Autodesk Fusion 360 part; units mm, degrees
(part 2 of 4)
  spline S9 degree 5 poles (13.0961, -23.3608) (13.1029, -23.373) (13.1162, -23.3975) (13.1351, -23.4347) (13.1584, -23.4852) (13.1848, -23.5497) (13.2094, -23.6151) (13.2328, -23.6811) (13.2556, -23.7474) (13.278, -23.814) (13.2999, -23.8807) (13.3212, -23.9477) (13.3416, -24.0151) (13.3612, -24.083) (13.3798, -24.1512) (13.3976, -24.2198) (13.4146, -24.2888) (13.4309, -24.358) (13.4467, -24.4275) (13.462, -24.4971) (13.4768, -24.567) (13.491, -24.6371) (13.5047, -24.7074) (13.5177, -24.778) (13.5302, -24.8488) (13.5421, -24.9198) (13.5534, -24.991) (13.5642, -25.0625) (13.5746, -25.1341) (13.5844, -25.2058) (13.5938, -25.2778) (13.6026, -25.3499) (13.611, -25.4222) (13.6189, -25.4947) (13.6263, -25.5673) (13.6332, -25.6401) (13.6397, -25.713) (13.6457, -25.7861) (13.6512, -25.8594) (13.6563, -25.9328) (13.661, -26.0063) (13.6652, -26.0799) (13.669, -26.1537) (13.6723, -26.2276) (13.6753, -26.3017) (13.6777, -26.3759) (13.6798, -26.4502) (13.6814, -26.5246) (13.6826, -26.5991) (13.6834, -26.6737) (13.6838, -26.7485) (13.6838, -26.8234) (13.6834, -26.8983) (13.6825, -26.9734) (13.6813, -27.0486) (13.6796, -27.1238) (13.6776, -27.1992) (13.6751, -27.2747) (13.6723, -27.3502) (13.6691, -27.4259) (13.6655, -27.5016) (13.6615, -27.5774) (13.6571, -27.6533) (13.6523, -27.7293) (13.6472, -27.8054) (13.6416, -27.8815) (13.6357, -27.9577) (13.6294, -28.034) (13.6228, -28.1104) (13.6157, -28.1868) (13.6083, -28.2633) (13.6021, -28.3246) (13.5973, -28.3705) (13.594, -28.4012) (13.5923, -28.4165) knots 0 0 0 0 0 0 0.01428571 0.02857143 0.04285714 0.05714286 0.07142857 0.08571429 0.1 0.11428571 0.12857143 0.14285714 0.15714286 0.17142857 0.18571429 0.2 0.21428571 0.22857143 0.24285714 0.25714286 0.27142857 0.28571429 0.3 0.31428571 0.32857143 0.34285714 0.35714286 0.37142857 0.38571429 0.4 0.41428571 0.42857143 0.44285714 0.45714286 0.47142857 0.48571429 0.5 0.51428571 0.52857143 0.54285714 0.55714286 0.57142857 0.58571429 0.6 0.61428571 0.62857143 0.64285714 0.65714286 0.67142857 0.68571429 0.7 0.71428571 0.72857143 0.74285714 0.75714286 0.77142857 0.78571429 0.8 0.81428571 0.82857143 0.84285714 0.85714286 0.87142857 0.88571429 0.9 0.91428571 0.92857143 0.94285714 0.95714286 0.97142857 0.98571429 1 1 1 1 1 1
  line L9 (13.0961, -23.3608) -> (12.631, -22.5302)
  arc A19 (12.9811, -21.189) -> (12.631, -22.5302) centre (13.5035, -22.0417) ccw
  arc A20 (12.9811, -21.189) -> (14.1898, -20.3993) centre (0, 0) ccw
  arc A21 (15.5588, -20.6174) -> (14.1898, -20.3993) centre (14.7609, -21.2202) ccw
  line L10 (15.5588, -20.6174) -> (16.1326, -21.377)
  spline S10 degree 5 poles (16.1326, -21.377) (16.141, -21.3881) (16.1581, -21.4101) (16.1845, -21.4424) (16.2215, -21.484) (16.2699, -21.5341) (16.3199, -21.5829) (16.371, -21.6309) (16.4225, -21.6784) (16.4745, -21.7256) (16.5268, -21.7724) (16.5797, -21.8189) (16.6332, -21.8647) (16.6874, -21.9098) (16.7424, -21.9543) (16.7981, -21.9981) (16.8545, -22.0414) (16.9113, -22.0842) (16.9685, -22.1266) (17.0262, -22.1686) (17.0842, -22.2102) (17.1427, -22.2513) (17.2016, -22.2921) (17.261, -22.3324) (17.3208, -22.3722) (17.3811, -22.4116) (17.4418, -22.4506) (17.5028, -22.4892) (17.5643, -22.5275) (17.626, -22.5653) (17.6882, -22.6028) (17.7507, -22.6399) (17.8135, -22.6766) (17.8767, -22.7129) (17.9402, -22.7489) (18.0041, -22.7845) (18.0683, -22.8197) (18.1328, -22.8545) (18.1977, -22.889) (18.2628, -22.9232) (18.3283, -22.957) (18.3941, -22.9904) (18.4601, -23.0235) (18.5265, -23.0563) (18.5931, -23.0887) (18.66, -23.1208) (18.7272, -23.1525) (18.7947, -23.1839) (18.8625, -23.2149) (18.9305, -23.2456) (18.9988, -23.276) (19.0674, -23.3061) (19.1362, -23.3358) (19.2053, -23.3652) (19.2746, -23.3942) (19.3442, -23.423) (19.4141, -23.4514) (19.4842, -23.4794) (19.5545, -23.5072) (19.6251, -23.5346) (19.6959, -23.5617) (19.7669, -23.5885) (19.8382, -23.615) (19.9097, -23.6412) (19.9814, -23.667) (20.0534, -23.6925) (20.1255, -23.7177) (20.1979, -23.7426) (20.2705, -23.7672) (20.3433, -23.7914) (20.4164, -23.8154) (20.475, -23.8343) (20.519, -23.8483) (20.5484, -23.8576) (20.5631, -23.8623) knots 0 0 0 0 0 0 0.01428571 0.02857143 0.04285714 0.05714286 0.07142857 0.08571429 0.1 0.11428571 0.12857143 0.14285714 0.15714286 0.17142857 0.18571429 0.2 0.21428571 0.22857143 0.24285714 0.25714286 0.27142857 0.28571429 0.3 0.31428571 0.32857143 0.34285714 0.35714286 0.37142857 0.38571429 0.4 0.41428571 0.42857143 0.44285714 0.45714286 0.47142857 0.48571429 0.5 0.51428571 0.52857143 0.54285714 0.55714286 0.57142857 0.58571429 0.6 0.61428571 0.62857143 0.64285714 0.65714286 0.67142857 0.68571429 0.7 0.71428571 0.72857143 0.74285714 0.75714286 0.77142857 0.78571429 0.8 0.81428571 0.82857143 0.84285714 0.85714286 0.87142857 0.88571429 0.9 0.91428571 0.92857143 0.94285714 0.95714286 0.97142857 0.98571429 1 1 1 1 1 1
  arc A22 (20.5631, -23.8623) -> (22.0827, -22.4634) centre (0, 0) ccw
  spline S11 degree 5 poles (19.9717, -17.8428) (19.9821, -17.8521) (20.0026, -17.8709) (20.0326, -17.9) (20.071, -17.9402) (20.117, -17.9926) (20.1615, -18.0465) (20.2051, -18.1013) (20.2482, -18.1566) (20.2909, -18.2123) (20.3333, -18.2683) (20.3752, -18.3248) (20.4165, -18.3819) (20.457, -18.4397) (20.4967, -18.4982) (20.5358, -18.5574) (20.5743, -18.6171) (20.6122, -18.6772) (20.6497, -18.7378) (20.6868, -18.7987) (20.7235, -18.86) (20.7597, -18.9217) (20.7955, -18.9837) (20.8307, -19.0463) (20.8655, -19.1092) (20.8998, -19.1725) (20.9336, -19.2362) (20.9671, -19.3002) (21.0001, -19.3646) (21.0327, -19.4293) (21.0649, -19.4943) (21.0967, -19.5596) (21.1281, -19.6253) (21.1591, -19.6913) (21.1897, -19.7576) (21.2199, -19.8241) (21.2497, -19.891) (21.2791, -19.9582) (21.3081, -20.0257) (21.3368, -20.0934) (21.365, -20.1615) (21.3929, -20.2298) (21.4205, -20.2983) (21.4476, -20.3672) (21.4744, -20.4362) (21.5009, -20.5056) (21.5269, -20.5752) (21.5526, -20.645) (21.578, -20.7151) (21.603, -20.7855) (21.6276, -20.8561) (21.6519, -20.9269) (21.6758, -20.9979) (21.6994, -21.0692) (21.7226, -21.1407) (21.7455, -21.2124) (21.7681, -21.2844) (21.7903, -21.3565) (21.8121, -21.4289) (21.8336, -21.5015) (21.8548, -21.5743) (21.8756, -21.6473) (21.8961, -21.7205) (21.9163, -21.7939) (21.9361, -21.8676) (21.9556, -21.9414) (21.9748, -22.0154) (21.9936, -22.0896) (22.0121, -22.164) (22.0302, -22.2385) (22.0481, -22.3133) (22.0621, -22.3733) (22.0724, -22.4183) (22.0793, -22.4484) (22.0827, -22.4634) knots 0 0 0 0 0 0 0.01428571 0.02857143 0.04285714 0.05714286 0.07142857 0.08571429 0.1 0.11428571 0.12857143 0.14285714 0.15714286 0.17142857 0.18571429 0.2 0.21428571 0.22857143 0.24285714 0.25714286 0.27142857 0.28571429 0.3 0.31428571 0.32857143 0.34285714 0.35714286 0.37142857 0.38571429 0.4 0.41428571 0.42857143 0.44285714 0.45714286 0.47142857 0.48571429 0.5 0.51428571 0.52857143 0.54285714 0.55714286 0.57142857 0.58571429 0.6 0.61428571 0.62857143 0.64285714 0.65714286 0.67142857 0.68571429 0.7 0.71428571 0.72857143 0.74285714 0.75714286 0.77142857 0.78571429 0.8 0.81428571 0.82857143 0.84285714 0.85714286 0.87142857 0.88571429 0.9 0.91428571 0.92857143 0.94285714 0.95714286 0.97142857 0.98571429 1 1 1 1 1 1
  line L11 (19.9717, -17.8428) -> (19.2622, -17.2082)
  arc A23 (19.1578, -15.8259) -> (19.2622, -17.2082) centre (19.9288, -16.4628) ccw
  arc A24 (19.1578, -15.8259) -> (20.0446, -14.6866) centre (0, 0) ccw
  arc A25 (21.4102, -14.4484) -> (20.0446, -14.6866) centre (20.8513, -15.2776) ccw
  line L12 (21.4102, -14.4484) -> (22.1996, -14.9805)
  spline S12 degree 5 poles (22.1996, -14.9805) (22.2111, -14.9883) (22.2344, -15.0035) (22.2699, -15.0254) (22.3184, -15.0528) (22.3805, -15.0845) (22.4436, -15.1144) (22.5075, -15.1432) (22.5717, -15.1714) (22.6361, -15.1992) (22.7008, -15.2265) (22.7659, -15.2532) (22.8314, -15.2792) (22.8974, -15.3043) (22.9638, -15.3285) (23.0308, -15.3519) (23.0981, -15.3745) (23.1657, -15.3965) (23.2336, -15.418) (23.3018, -15.439) (23.3702, -15.4595) (23.4389, -15.4795) (23.5078, -15.4989) (23.5771, -15.5177) (23.6466, -15.536) (23.7164, -15.5537) (23.7864, -15.5709) (23.8567, -15.5876) (23.9272, -15.6038) (23.998, -15.6195) (24.0689, -15.6348) (24.14, -15.6495) (24.2114, -15.6639) (24.283, -15.6777) (24.3547, -15.6911) (24.4267, -15.704) (24.4989, -15.7165) (24.5712, -15.7285) (24.6437, -15.7401) (24.7165, -15.7512) (24.7893, -15.7619) (24.8624, -15.7722) (24.9356, -15.7821) (25.009, -15.7915) (25.0826, -15.8005) (25.1563, -15.8091) (25.2302, -15.8173) (25.3042, -15.8251) (25.3783, -15.8324) (25.4527, -15.8394) (25.5271, -15.8459) (25.6017, -15.8521) (25.6765, -15.8579) (25.7514, -15.8632) (25.8264, -15.8682) (25.9015, -15.8728) (25.9768, -15.877) (26.0522, -15.8808) (26.1277, -15.8842) (26.2034, -15.8872) (26.2792, -15.8899) (26.3551, -15.8921) (26.4311, -15.894) (26.5072, -15.8956) (26.5834, -15.8967) (26.6598, -15.8975) (26.7362, -15.8979) (26.8127, -15.8979) (26.8894, -15.8976) (26.9662, -15.8969) (27.043, -15.8958) (27.1046, -15.8947) (27.1508, -15.8936) (27.1816, -15.8929) (27.197, -15.8925) knots 0 0 0 0 0 0 0.01428571 0.02857143 0.04285714 0.05714286 0.07142857 0.08571429 0.1 0.11428571 0.12857143 0.14285714 0.15714286 0.17142857 0.18571429 0.2 0.21428571 0.22857143 0.24285714 0.25714286 0.27142857 0.28571429 0.3 0.31428571 0.32857143 0.34285714 0.35714286 0.37142857 0.38571429 0.4 0.41428571 0.42857143 0.44285714 0.45714286 0.47142857 0.48571429 0.5 0.51428571 0.52857143 0.54285714 0.55714286 0.57142857 0.58571429 0.6 0.61428571 0.62857143 0.64285714 0.65714286 0.67142857 0.68571429 0.7 0.71428571 0.72857143 0.74285714 0.75714286 0.77142857 0.78571429 0.8 0.81428571 0.82857143 0.84285714 0.85714286 0.87142857 0.88571429 0.9 0.91428571 0.92857143 0.94285714 0.95714286 0.97142857 0.98571429 1 1 1 1 1 1
  arc A26 (27.197, -15.8925) -> (28.18, -14.0761) centre (0, 0) ccw
  spline S13 degree 5 poles (24.6832, -10.3912) (24.696, -10.3966) (24.7215, -10.4078) (24.7593, -10.4255) (24.8087, -10.4511) (24.8692, -10.4857) (24.9288, -10.5222) (24.9878, -10.5599) (25.0465, -10.5983) (25.105, -10.6371) (25.1633, -10.6763) (25.2213, -10.7161) (25.2788, -10.7567) (25.3359, -10.7982) (25.3925, -10.8407) (25.4487, -10.8839) (25.5045, -10.9279) (25.5599, -10.9725) (25.615, -11.0175) (25.6699, -11.0631) (25.7245, -11.1092) (25.7787, -11.1558) (25.8327, -11.2029) (25.8863, -11.2506) (25.9397, -11.2988) (25.9927, -11.3475) (26.0454, -11.3968) (26.0978, -11.4465) (26.1499, -11.4966) (26.2018, -11.5472) (26.2533, -11.5983) (26.3046, -11.6497) (26.3556, -11.7016) (26.4064, -11.754) (26.4568, -11.8068) (26.507, -11.8599) (26.5569, -11.9135) (26.6065, -11.9675) (26.6559, -12.0219) (26.705, -12.0767) (26.7538, -12.1318) (26.8024, -12.1874) (26.8507, -12.2433) (26.8988, -12.2996) (26.9465, -12.3562) (26.994, -12.4132) (27.0413, -12.4706) (27.0883, -12.5283) (27.135, -12.5864) (27.1815, -12.6448) (27.2277, -12.7035) (27.2737, -12.7626) (27.3194, -12.8221) (27.3648, -12.8818) (27.41, -12.9419) (27.455, -13.0023) (27.4996, -13.063) (27.5441, -13.1241) (27.5882, -13.1855) (27.6321, -13.2471) (27.6758, -13.3091) (27.7192, -13.3714) (27.7624, -13.434) (27.8053, -13.4969) (27.8479, -13.5601) (27.8903, -13.6236) (27.9325, -13.6873) (27.9744, -13.7514) (28.016, -13.8158) (28.0574, -13.8804) (28.0986, -13.9453) (28.1313, -13.9975) (28.1557, -14.0367) (28.1719, -14.063) (28.18, -14.0761) knots 0 0 0 0 0 0 0.01428571 0.02857143 0.04285714 0.05714286 0.07142857 0.08571429 0.1 0.11428571 0.12857143 0.14285714 0.15714286 0.17142857 0.18571429 0.2 0.21428571 0.22857143 0.24285714 0.25714286 0.27142857 0.28571429 0.3 0.31428571 0.32857143 0.34285714 0.35714286 0.37142857 0.38571429 0.4 0.41428571 0.42857143 0.44285714 0.45714286 0.47142857 0.48571429 0.5 0.51428571 0.52857143 0.54285714 0.55714286 0.57142857 0.58571429 0.6 0.61428571 0.62857143 0.64285714 0.65714286 0.67142857 0.68571429 0.7 0.71428571 0.72857143 0.74285714 0.75714286 0.77142857 0.78571429 0.8 0.81428571 0.82857143 0.84285714 0.85714286 0.87142857 0.88571429 0.9 0.91428571 0.92857143 0.94285714 0.95714286 0.97142857 0.98571429 1 1 1 1 1 1
  line L13 (24.6832, -10.3912) -> (23.806, -10.0214)
  arc A27 (23.2585, -8.7479) -> (23.806, -10.0214) centre (24.1945, -9.0999) ccw
  arc A28 (23.2585, -8.7479) -> (23.7273, -7.3823) centre (0, 0) ccw
  arc A29 (24.9416, -6.7137) -> (23.7273, -7.3823) centre (24.6821, -7.6794) ccw
  line L14 (24.9416, -6.7137) -> (25.8609, -6.9606)
  spline S14 degree 5 poles (25.8609, -6.9606) (25.8743, -6.9642) (25.9013, -6.9711) (25.942, -6.9803) (25.9968, -6.9904) (26.0658, -7.0003) (26.1352, -7.008) (26.2049, -7.0145) (26.2748, -7.0204) (26.3448, -7.0257) (26.4149, -7.0305) (26.4851, -7.0347) (26.5555, -7.038) (26.626, -7.0403) (26.6967, -7.0416) (26.7676, -7.042) (26.8386, -7.0415) (26.9098, -7.0404) (26.981, -7.0387) (27.0523, -7.0364) (27.1236, -7.0336) (27.1951, -7.0302) (27.2666, -7.0261) (27.3382, -7.0215) (27.4099, -7.0161) (27.4817, -7.0102) (27.5535, -7.0037) (27.6254, -6.9967) (27.6973, -6.9891) (27.7693, -6.9811) (27.8414, -6.9725) (27.9135, -6.9634) (27.9856, -6.9537) (28.0578, -6.9436) (28.13, -6.9329) (28.2023, -6.9218) (28.2746, -6.9101) (28.3469, -6.898) (28.4193, -6.8854) (28.4917, -6.8723) (28.5641, -6.8588) (28.6365, -6.8448) (28.709, -6.8304) (28.7814, -6.8155) (28.8539, -6.8001) (28.9265, -6.7843) (28.999, -6.7681) (29.0715, -6.7514) (29.1441, -6.7343) (29.2166, -6.7167) (29.2892, -6.6987) (29.3617, -6.6803) (29.4343, -6.6615) (29.5069, -6.6423) (29.5794, -6.6226) (29.652, -6.6025) (29.7246, -6.582) (29.7971, -6.5612) (29.8697, -6.5399) (29.9422, -6.5182) (30.0147, -6.4961) (30.0872, -6.4736) (30.1597, -6.4507) (30.2322, -6.4274) (30.3047, -6.4038) (30.3772, -6.3797) (30.4496, -6.3553) (30.522, -6.3304) (30.5944, -6.3052) (30.6668, -6.2796) (30.7391, -6.2537) (30.797, -6.2326) (30.8403, -6.2166) (30.8693, -6.2059) (30.8837, -6.2005) knots 0 0 0 0 0 0 0.01428571 0.02857143 0.04285714 0.05714286 0.07142857 0.08571429 0.1 0.11428571 0.12857143 0.14285714 0.15714286 0.17142857 0.18571429 0.2 0.21428571 0.22857143 0.24285714 0.25714286 0.27142857 0.28571429 0.3 0.31428571 0.32857143 0.34285714 0.35714286 0.37142857 0.38571429 0.4 0.41428571 0.42857143 0.44285714 0.45714286 0.47142857 0.48571429 0.5 0.51428571 0.52857143 0.54285714 0.55714286 0.57142857 0.58571429 0.6 0.61428571 0.62857143 0.64285714 0.65714286 0.67142857 0.68571429 0.7 0.71428571 0.72857143 0.74285714 0.75714286 0.77142857 0.78571429 0.8 0.81428571 0.82857143 0.84285714 0.85714286 0.87142857 0.88571429 0.9 0.91428571 0.92857143 0.94285714 0.95714286 0.97142857 0.98571429 1 1 1 1 1 1
  arc A30 (30.8837, -6.2005) -> (31.2237, -4.1634) centre (0, 0) ccw
  spline S15 degree 5 poles (26.7198, -1.8136) (26.7337, -1.8145) (26.7614, -1.8168) (26.8029, -1.8213) (26.858, -1.8295) (26.9264, -1.8426) (26.9947, -1.8578) (27.0627, -1.8742) (27.1307, -1.8914) (27.1986, -1.9091) (27.2665, -1.9273) (27.3342, -1.9461) (27.4019, -1.9659) (27.4693, -1.9866) (27.5366, -2.0083) (27.6038, -2.031) (27.6708, -2.0545) (27.7377, -2.0787) (27.8045, -2.1034) (27.8712, -2.1287) (27.9378, -2.1545) (28.0043, -2.181) (28.0706, -2.208) (28.1368, -2.2357) (28.2029, -2.264) (28.2688, -2.2929) (28.3347, -2.3223) (28.4004, -2.3523) (28.466, -2.3829) (28.5315, -2.4139) (28.5968, -2.4454) (28.662, -2.4774) (28.7271, -2.51) (28.7921, -2.543) (28.857, -2.5765) (28.9217, -2.6105) (28.9863, -2.645) (29.0508, -2.68) (29.1151, -2.7154) (29.1794, -2.7512) (29.2434, -2.7876) (29.3074, -2.8243) (29.3713, -2.8615) (29.435, -2.8991) (29.4986, -2.9372) (29.562, -2.9757) (29.6253, -3.0146) (29.6885, -3.0539) (29.7516, -3.0937) (29.8145, -3.1338) (29.8773, -3.1744) (29.9399, -3.2154) (30.0025, -3.2567) (30.0648, -3.2985) (30.1271, -3.3407) (30.1892, -3.3832) (30.2512, -3.4261) (30.313, -3.4695) (30.3747, -3.5131) (30.4363, -3.5572) (30.4977, -3.6017) (30.559, -3.6465) (30.6201, -3.6917) (30.6811, -3.7372) (30.742, -3.7831) (30.8027, -3.8294) (30.8633, -3.8761) (30.9237, -3.923) (30.984, -3.9704) (31.0441, -4.0181) (31.1041, -4.0661) (31.152, -4.1049) (31.1879, -4.134) (31.2117, -4.1536) (31.2237, -4.1634) knots 0 0 0 0 0 0 0.01428571 0.02857143 0.04285714 0.05714286 0.07142857 0.08571429 0.1 0.11428571 0.12857143 0.14285714 0.15714286 0.17142857 0.18571429 0.2 0.21428571 0.22857143 0.24285714 0.25714286 0.27142857 0.28571429 0.3 0.31428571 0.32857143 0.34285714 0.35714286 0.37142857 0.38571429 0.4 0.41428571 0.42857143 0.44285714 0.45714286 0.47142857 0.48571429 0.5 0.51428571 0.52857143 0.54285714 0.55714286 0.57142857 0.58571429 0.6 0.61428571 0.62857143 0.64285714 0.65714286 0.67142857 0.68571429 0.7 0.71428571 0.72857143 0.74285714 0.75714286 0.77142857 0.78571429 0.8 0.81428571 0.82857143 0.84285714 0.85714286 0.87142857 0.88571429 0.9 0.91428571 0.92857143 0.94285714 0.95714286 0.97142857 0.98571429 1 1 1 1 1 1
  line L15 (26.7198, -1.8136) -> (25.7701, -1.7486)
  arc A31 (24.8387, -0.7219) -> (25.7701, -1.7486) centre (25.8383, -0.7509) ccw
  arc A32 (24.8387, -0.7219) -> (24.8387, 0.7219) centre (0, 0) ccw
  arc A33 (25.7701, 1.7486) -> (24.8387, 0.7219) centre (25.8383, 0.7509) ccw
  line L16 (25.7701, 1.7486) -> (26.7198, 1.8136)
  spline S16 degree 5 poles (26.7198, 1.8136) (26.7337, 1.8145) (26.7614, 1.8168) (26.8029, 1.8213) (26.858, 1.8295) (26.9264, 1.8426) (26.9947, 1.8578) (27.0627, 1.8742) (27.1307, 1.8914) (27.1986, 1.9091) (27.2665, 1.9273) (27.3342, 1.9461) (27.4019, 1.9659) (27.4693, 1.9866) (27.5366, 2.0083) (27.6038, 2.031) (27.6708, 2.0545) (27.7377, 2.0787) (27.8045, 2.1034) (27.8712, 2.1287) (27.9378, 2.1545) (28.0043, 2.181) (28.0706, 2.208) (28.1368, 2.2357) (28.2029, 2.264) (28.2688, 2.2929) (28.3347, 2.3223) (28.4004, 2.3523) (28.466, 2.3829) (28.5315, 2.4139) (28.5968, 2.4454) (28.662, 2.4774) (28.7271, 2.51) (28.7921, 2.543) (28.857, 2.5765) (28.9217, 2.6105) (28.9863, 2.645) (29.0508, 2.68) (29.1151, 2.7154) (29.1794, 2.7512) (29.2434, 2.7876) (29.3074, 2.8243) (29.3713, 2.8615) (29.435, 2.8991) (29.4986, 2.9372) (29.562, 2.9757) (29.6253, 3.0146) (29.6885, 3.0539) (29.7516, 3.0937) (29.8145, 3.1338) (29.8773, 3.1744) (29.9399, 3.2154) (30.0025, 3.2567) (30.0648, 3.2985) (30.1271, 3.3407) (30.1892, 3.3832) (30.2512, 3.4261) (30.313, 3.4695) (30.3747, 3.5131) (30.4363, 3.5572) (30.4977, 3.6017) (30.559, 3.6465) (30.6201, 3.6917) (30.6811, 3.7372) (30.742, 3.7831) (30.8027, 3.8294) (30.8633, 3.8761) (30.9237, 3.923) (30.984, 3.9704) (31.0441, 4.0181) (31.1041, 4.0661) (31.152, 4.1049) (31.1879, 4.134) (31.2117, 4.1536) (31.2237, 4.1634) knots 0 0 0 0 0 0 0.01428571 0.02857143 0.04285714 0.05714286 0.07142857 0.08571429 0.1 0.11428571 0.12857143 0.14285714 0.15714286 0.17142857 0.18571429 0.2 0.21428571 0.22857143 0.24285714 0.25714286 0.27142857 0.28571429 0.3 0.31428571 0.32857143 0.34285714 0.35714286 0.37142857 0.38571429 0.4 0.41428571 0.42857143 0.44285714 0.45714286 0.47142857 0.48571429 0.5 0.51428571 0.52857143 0.54285714 0.55714286 0.57142857 0.58571429 0.6 0.61428571 0.62857143 0.64285714 0.65714286 0.67142857 0.68571429 0.7 0.71428571 0.72857143 0.74285714 0.75714286 0.77142857 0.78571429 0.8 0.81428571 0.82857143 0.84285714 0.85714286 0.87142857 0.88571429 0.9 0.91428571 0.92857143 0.94285714 0.95714286 0.97142857 0.98571429 1 1 1 1 1 1
  arc A34 (31.2237, 4.1634) -> (30.8837, 6.2005) centre (0, 0) ccw
  spline S17 degree 5 poles (25.8609, 6.9606) (25.8743, 6.9642) (25.9013, 6.9711) (25.942, 6.9803) (25.9968, 6.9904) (26.0658, 7.0003) (26.1352, 7.008) (26.2049, 7.0145) (26.2748, 7.0204) (26.3448, 7.0257) (26.4149, 7.0305) (26.4851, 7.0347) (26.5555, 7.038) (26.626, 7.0403) (26.6967, 7.0416) (26.7676, 7.042) (26.8386, 7.0415) (26.9098, 7.0404) (26.981, 7.0387) (27.0523, 7.0364) (27.1236, 7.0336) (27.1951, 7.0302) (27.2666, 7.0261) (27.3382, 7.0215) (27.4099, 7.0161) (27.4817, 7.0102) (27.5535, 7.0037) (27.6254, 6.9967) (27.6973, 6.9891) (27.7693, 6.9811) (27.8414, 6.9725) (27.9135, 6.9634) (27.9856, 6.9537) (28.0578, 6.9436) (28.13, 6.9329) (28.2023, 6.9218) (28.2746, 6.9101) (28.3469, 6.898) (28.4193, 6.8854) (28.4917, 6.8723) (28.5641, 6.8588) (28.6365, 6.8448) (28.709, 6.8304) (28.7814, 6.8155) (28.8539, 6.8001) (28.9265, 6.7843) (28.999, 6.7681) (29.0715, 6.7514) (29.1441, 6.7343) (29.2166, 6.7167) (29.2892, 6.6987) (29.3617, 6.6803) (29.4343, 6.6615) (29.5069, 6.6423) (29.5794, 6.6226) (29.652, 6.6025) (29.7246, 6.582) (29.7971, 6.5612) (29.8697, 6.5399) (29.9422, 6.5182) (30.0147, 6.4961) (30.0872, 6.4736) (30.1597, 6.4507) (30.2322, 6.4274) (30.3047, 6.4038) (30.3772, 6.3797) (30.4496, 6.3553) (30.522, 6.3304) (30.5944, 6.3052) (30.6668, 6.2796) (30.7391, 6.2537) (30.797, 6.2326) (30.8403, 6.2166) (30.8693, 6.2059) (30.8837, 6.2005) knots 0 0 0 0 0 0 0.01428571 0.02857143 0.04285714 0.05714286 0.07142857 0.08571429 0.1 0.11428571 0.12857143 0.14285714 0.15714286 0.17142857 0.18571429 0.2 0.21428571 0.22857143 0.24285714 0.25714286 0.27142857 0.28571429 0.3 0.31428571 0.32857143 0.34285714 0.35714286 0.37142857 0.38571429 0.4 0.41428571 0.42857143 0.44285714 0.45714286 0.47142857 0.48571429 0.5 0.51428571 0.52857143 0.54285714 0.55714286 0.57142857 0.58571429 0.6 0.61428571 0.62857143 0.64285714 0.65714286 0.67142857 0.68571429 0.7 0.71428571 0.72857143 0.74285714 0.75714286 0.77142857 0.78571429 0.8 0.81428571 0.82857143 0.84285714 0.85714286 0.87142857 0.88571429 0.9 0.91428571 0.92857143 0.94285714 0.95714286 0.97142857 0.98571429 1 1 1 1 1 1
  line L17 (25.8609, 6.9606) -> (24.9416, 6.7137)
  arc A35 (23.7273, 7.3823) -> (24.9416, 6.7137) centre (24.6821, 7.6794) ccw
  arc A36 (23.7273, 7.3823) -> (23.2585, 8.7479) centre (0, 0) ccw
  arc A37 (23.806, 10.0214) -> (23.2585, 8.7479) centre (24.1945, 9.0999) ccw
  line L18 (23.806, 10.0214) -> (24.6832, 10.3912)
  spline S18 degree 5 poles (24.6832, 10.3912) (24.696, 10.3966) (24.7215, 10.4078) (24.7593, 10.4255) (24.8087, 10.4511) (24.8692, 10.4857) (24.9288, 10.5222) (24.9878, 10.5599) (25.0465, 10.5983) (25.105, 10.6371) (25.1633, 10.6763) (25.2213, 10.7161) (25.2788, 10.7567) (25.3359, 10.7982) (25.3925, 10.8407) (25.4487, 10.8839) (25.5045, 10.9279) (25.5599, 10.9725) (25.615, 11.0175) (25.6699, 11.0631) (25.7245, 11.1092) (25.7787, 11.1558) (25.8327, 11.2029) (25.8863, 11.2506) (25.9397, 11.2988) (25.9927, 11.3475) (26.0454, 11.3968) (26.0978, 11.4465) (26.1499, 11.4966) (26.2018, 11.5472) (26.2533, 11.5983) (26.3046, 11.6497) (26.3556, 11.7016) (26.4064, 11.754) (26.4568, 11.8068) (26.507, 11.8599) (26.5569, 11.9135) (26.6065, 11.9675) (26.6559, 12.0219) (26.705, 12.0767) (26.7538, 12.1318) (26.8024, 12.1874) (26.8507, 12.2433) (26.8988, 12.2996) (26.9465, 12.3562) (26.994, 12.4132) (27.0413, 12.4706) (27.0883, 12.5283) (27.135, 12.5864) (27.1815, 12.6448) (27.2277, 12.7035) (27.2737, 12.7626) (27.3194, 12.8221) (27.3648, 12.8818) (27.41, 12.9419) (27.455, 13.0023) (27.4996, 13.063) (27.5441, 13.1241) (27.5882, 13.1855) (27.6321, 13.2471) (27.6758, 13.3091) (27.7192, 13.3714) (27.7624, 13.434) (27.8053, 13.4969) (27.8479, 13.5601) (27.8903, 13.6236) (27.9325, 13.6873) (27.9744, 13.7514) (28.016, 13.8158) (28.0574, 13.8804) (28.0986, 13.9453) (28.1313, 13.9975) (28.1557, 14.0367) (28.1719, 14.063) (28.18, 14.0761) knots 0 0 0 0 0 0 0.01428571 0.02857143 0.04285714 0.05714286 0.07142857 0.08571429 0.1 0.11428571 0.12857143 0.14285714 0.15714286 0.17142857 0.18571429 0.2 0.21428571 0.22857143 0.24285714 0.25714286 0.27142857 0.28571429 0.3 0.31428571 0.32857143 0.34285714 0.35714286 0.37142857 0.38571429 0.4 0.41428571 0.42857143 0.44285714 0.45714286 0.47142857 0.48571429 0.5 0.51428571 0.52857143 0.54285714 0.55714286 0.57142857 0.58571429 0.6 0.61428571 0.62857143 0.64285714 0.65714286 0.67142857 0.68571429 0.7 0.71428571 0.72857143 0.74285714 0.75714286 0.77142857 0.78571429 0.8 0.81428571 0.82857143 0.84285714 0.85714286 0.87142857 0.88571429 0.9 0.91428571 0.92857143 0.94285714 0.95714286 0.97142857 0.98571429 1 1 1 1 1 1
  arc A38 (28.18, 14.0761) -> (27.197, 15.8925) centre (0, 0) ccw
  spline S19 degree 5 poles (22.1996, 14.9805) (22.2111, 14.9883) (22.2344, 15.0035) (22.2699, 15.0254) (22.3184, 15.0528) (22.3805, 15.0845) (22.4436, 15.1144) (22.5075, 15.1432) (22.5717, 15.1714) (22.6361, 15.1992) (22.7008, 15.2265) (22.7659, 15.2532) (22.8314, 15.2792) (22.8974, 15.3043) (22.9638, 15.3285) (23.0308, 15.3519) (23.0981, 15.3745) (23.1657, 15.3965) (23.2336, 15.418) (23.3018, 15.439) (23.3702, 15.4595) (23.4389, 15.4795) (23.5078, 15.4989) (23.5771, 15.5177) (23.6466, 15.536) (23.7164, 15.5537) (23.7864, 15.5709) (23.8567, 15.5876) (23.9272, 15.6038) (23.998, 15.6195) (24.0689, 15.6348) (24.14, 15.6495) (24.2114, 15.6639) (24.283, 15.6777) (24.3547, 15.6911) (24.4267, 15.704) (24.4989, 15.7165) (24.5712, 15.7285) (24.6437, 15.7401) (24.7165, 15.7512) (24.7893, 15.7619) (24.8624, 15.7722) (24.9356, 15.7821) (25.009, 15.7915) (25.0826, 15.8005) (25.1563, 15.8091) (25.2302, 15.8173) (25.3042, 15.8251) (25.3783, 15.8324) (25.4527, 15.8394) (25.5271, 15.8459) (25.6017, 15.8521) (25.6765, 15.8579) (25.7514, 15.8632) (25.8264, 15.8682) (25.9015, 15.8728) (25.9768, 15.877) (26.0522, 15.8808) (26.1277, 15.8842) (26.2034, 15.8872) (26.2792, 15.8899) (26.3551, 15.8921) (26.4311, 15.894) (26.5072, 15.8956) (26.5834, 15.8967) (26.6598, 15.8975) (26.7362, 15.8979) (26.8127, 15.8979) (26.8894, 15.8976) (26.9662, 15.8969) (27.043, 15.8958) (27.1046, 15.8947) (27.1508, 15.8936) (27.1816, 15.8929) (27.197, 15.8925) knots 0 0 0 0 0 0 0.01428571 0.02857143 0.04285714 0.05714286 0.07142857 0.08571429 0.1 0.11428571 0.12857143 0.14285714 0.15714286 0.17142857 0.18571429 0.2 0.21428571 0.22857143 0.24285714 0.25714286 0.27142857 0.28571429 0.3 0.31428571 0.32857143 0.34285714 0.35714286 0.37142857 0.38571429 0.4 0.41428571 0.42857143 0.44285714 0.45714286 0.47142857 0.48571429 0.5 0.51428571 0.52857143 0.54285714 0.55714286 0.57142857 0.58571429 0.6 0.61428571 0.62857143 0.64285714 0.65714286 0.67142857 0.68571429 0.7 0.71428571 0.72857143 0.74285714 0.75714286 0.77142857 0.78571429 0.8 0.81428571 0.82857143 0.84285714 0.85714286 0.87142857 0.88571429 0.9 0.91428571 0.92857143 0.94285714 0.95714286 0.97142857 0.98571429 1 1 1 1 1 1
  line L19 (22.1996, 14.9805) -> (21.4102, 14.4484)
  arc A39 (20.0446, 14.6866) -> (21.4102, 14.4484) centre (20.8513, 15.2776) ccw
  arc A40 (20.0446, 14.6866) -> (19.1578, 15.8259) centre (0, 0) ccw
  arc A41 (19.2622, 17.2082) -> (19.1578, 15.8259) centre (19.9288, 16.4628) ccw
  line L20 (19.2622, 17.2082) -> (19.9717, 17.8428)
  spline S20 degree 5 poles (19.9717, 17.8428) (19.9821, 17.8521) (20.0026, 17.8709) (20.0326, 17.9) (20.071, 17.9402) (20.117, 17.9926) (20.1615, 18.0465) (20.2051, 18.1013) (20.2482, 18.1566) (20.2909, 18.2123) (20.3333, 18.2683) (20.3752, 18.3248) (20.4165, 18.3819) (20.457, 18.4397) (20.4967, 18.4982) (20.5358, 18.5574) (20.5743, 18.6171) (20.6122, 18.6772) (20.6497, 18.7378) (20.6868, 18.7987) (20.7235, 18.86) (20.7597, 18.9217) (20.7955, 18.9837) (20.8307, 19.0463) (20.8655, 19.1092) (20.8998, 19.1725) (20.9336, 19.2362) (20.9671, 19.3002) (21.0001, 19.3646) (21.0327, 19.4293) (21.0649, 19.4943) (21.0967, 19.5596) (21.1281, 19.6253) (21.1591, 19.6913) (21.1897, 19.7576) (21.2199, 19.8241) (21.2497, 19.891) (21.2791, 19.9582) (21.3081, 20.0257) (21.3368, 20.0934) (21.365, 20.1615) (21.3929, 20.2298) (21.4205, 20.2983) (21.4476, 20.3672) (21.4744, 20.4362) (21.5009, 20.5056) (21.5269, 20.5752) (21.5526, 20.645) (21.578, 20.7151) (21.603, 20.7855) (21.6276, 20.8561) (21.6519, 20.9269) (21.6758, 20.9979) (21.6994, 21.0692) (21.7226, 21.1407) (21.7455, 21.2124) (21.7681, 21.2844) (21.7903, 21.3565) (21.8121, 21.4289) (21.8336, 21.5015) (21.8548, 21.5743) (21.8756, 21.6473) (21.8961, 21.7205) (21.9163, 21.7939) (21.9361, 21.8676) (21.9556, 21.9414) (21.9748, 22.0154) (21.9936, 22.0896) (22.0121, 22.164) (22.0302, 22.2385) (22.0481, 22.3133) (22.0621, 22.3733) (22.0724, 22.4183) (22.0793, 22.4484) (22.0827, 22.4634) knots 0 0 0 0 0 0 0.01428571 0.02857143 0.04285714 0.05714286 0.07142857 0.08571429 0.1 0.11428571 0.12857143 0.14285714 0.15714286 0.17142857 0.18571429 0.2 0.21428571 0.22857143 0.24285714 0.25714286 0.27142857 0.28571429 0.3 0.31428571 0.32857143 0.34285714 0.35714286 0.37142857 0.38571429 0.4 0.41428571 0.42857143 0.44285714 0.45714286 0.47142857 0.48571429 0.5 0.51428571 0.52857143 0.54285714 0.55714286 0.57142857 0.58571429 0.6 0.61428571 0.62857143 0.64285714 0.65714286 0.67142857 0.68571429 0.7 0.71428571 0.72857143 0.74285714 0.75714286 0.77142857 0.78571429 0.8 0.81428571 0.82857143 0.84285714 0.85714286 0.87142857 0.88571429 0.9 0.91428571 0.92857143 0.94285714 0.95714286 0.97142857 0.98571429 1 1 1 1 1 1
  arc A42 (22.0827, 22.4634) -> (20.5631, 23.8623) centre (0, 0) ccw
  spline S21 degree 5 poles (16.1326, 21.377) (16.141, 21.3881) (16.1581, 21.4101) (16.1845, 21.4424) (16.2215, 21.484) (16.2699, 21.5341) (16.3199, 21.5829) (16.371, 21.6309) (16.4225, 21.6784) (16.4745, 21.7256) (16.5268, 21.7724) (16.5797, 21.8189) (16.6332, 21.8647) (16.6874, 21.9098) (16.7424, 21.9543) (16.7981, 21.9981) (16.8545, 22.0414) (16.9113, 22.0842) (16.9685, 22.1266) (17.0262, 22.1686) (17.0842, 22.2102) (17.1427, 22.2513) (17.2016, 22.2921) (17.261, 22.3324) (17.3208, 22.3722) (17.3811, 22.4116) (17.4418, 22.4506) (17.5028, 22.4892) (17.5643, 22.5275) (17.626, 22.5653) (17.6882, 22.6028) (17.7507, 22.6399) (17.8135, 22.6766) (17.8767, 22.7129) (17.9402, 22.7489) (18.0041, 22.7845) (18.0683, 22.8197) (18.1328, 22.8545) (18.1977, 22.889) (18.2628, 22.9232) (18.3283, 22.957) (18.3941, 22.9904) (18.4601, 23.0235) (18.5265, 23.0563) (18.5931, 23.0887) (18.66, 23.1208) (18.7272, 23.1525) (18.7947, 23.1839) (18.8625, 23.2149) (18.9305, 23.2456) (18.9988, 23.276) (19.0674, 23.3061) (19.1362, 23.3358) (19.2053, 23.3652) (19.2746, 23.3942) (19.3442, 23.423) (19.4141, 23.4514) (19.4842, 23.4794) (19.5545, 23.5072) (19.6251, 23.5346) (19.6959, 23.5617) (19.7669, 23.5885) (19.8382, 23.615) (19.9097, 23.6412) (19.9814, 23.667) (20.0534, 23.6925) (20.1255, 23.7177) (20.1979, 23.7426) (20.2705, 23.7672) (20.3433, 23.7914) (20.4164, 23.8154) (20.475, 23.8343) (20.519, 23.8483) (20.5484, 23.8576) (20.5631, 23.8623) knots 0 0 0 0 0 0 0.01428571 0.02857143 0.04285714 0.05714286 0.07142857 0.08571429 0.1 0.11428571 0.12857143 0.14285714 0.15714286 0.17142857 0.18571429 0.2 0.21428571 0.22857143 0.24285714 0.25714286 0.27142857 0.28571429 0.3 0.31428571 0.32857143 0.34285714 0.35714286 0.37142857 0.38571429 0.4 0.41428571 0.42857143 0.44285714 0.45714286 0.47142857 0.48571429 0.5 0.51428571 0.52857143 0.54285714 0.55714286 0.57142857 0.58571429 0.6 0.61428571 0.62857143 0.64285714 0.65714286 0.67142857 0.68571429 0.7 0.71428571 0.72857143 0.74285714 0.75714286 0.77142857 0.78571429 0.8 0.81428571 0.82857143 0.84285714 0.85714286 0.87142857 0.88571429 0.9 0.91428571 0.92857143 0.94285714 0.95714286 0.97142857 0.98571429 1 1 1 1 1 1
  line L21 (16.1326, 21.377) -> (15.5588, 20.6174)
  arc A43 (14.1898, 20.3993) -> (15.5588, 20.6174) centre (14.7609, 21.2202) ccw
  arc A44 (14.1898, 20.3993) -> (12.9811, 21.189) centre (0, 0) ccw
  arc A45 (12.631, 22.5302) -> (12.9811, 21.189) centre (13.5035, 22.0417) ccw
  line L22 (12.631, 22.5302) -> (13.0961, 23.3608)
  spline S22 degree 5 poles (13.0961, 23.3608) (13.1029, 23.373) (13.1162, 23.3975) (13.1351, 23.4347) (13.1584, 23.4852) (13.1848, 23.5497) (13.2094, 23.6151) (13.2328, 23.6811) (13.2556, 23.7474) (13.278, 23.814) (13.2999, 23.8807) (13.3212, 23.9477) (13.3416, 24.0151) (13.3612, 24.083) (13.3798, 24.1512) (13.3976, 24.2198) (13.4146, 24.2888) (13.4309, 24.358) (13.4467, 24.4275) (13.462, 24.4971) (13.4768, 24.567) (13.491, 24.6371) (13.5047, 24.7074) (13.5177, 24.778) (13.5302, 24.8488) (13.5421, 24.9198) (13.5534, 24.991) (13.5642, 25.0625) (13.5746, 25.1341) (13.5844, 25.2058) (13.5938, 25.2778) (13.6026, 25.3499) (13.611, 25.4222) (13.6189, 25.4947) (13.6263, 25.5673) (13.6332, 25.6401) (13.6397, 25.713) (13.6457, 25.7861) (13.6512, 25.8594) (13.6563, 25.9328) (13.661, 26.0063) (13.6652, 26.0799) (13.669, 26.1537) (13.6723, 26.2276) (13.6753, 26.3017) (13.6777, 26.3759) (13.6798, 26.4502) (13.6814, 26.5246) (13.6826, 26.5991) (13.6834, 26.6737) (13.6838, 26.7485) (13.6838, 26.8234) (13.6834, 26.8983) (13.6825, 26.9734) (13.6813, 27.0486) (13.6796, 27.1238) (13.6776, 27.1992) (13.6751, 27.2747) (13.6723, 27.3502) (13.6691, 27.4259) (13.6655, 27.5016) (13.6615, 27.5774) (13.6571, 27.6533) (13.6523, 27.7293) (13.6472, 27.8054) (13.6416, 27.8815) (13.6357, 27.9577) (13.6294, 28.034) (13.6228, 28.1104) (13.6157, 28.1868) (13.6083, 28.2633) (13.6021, 28.3246) (13.5973, 28.3705) (13.594, 28.4012) (13.5923, 28.4165) knots 0 0 0 0 0 0 0.01428571 0.02857143 0.04285714 0.05714286 0.07142857 0.08571429 0.1 0.11428571 0.12857143 0.14285714 0.15714286 0.17142857 0.18571429 0.2 0.21428571 0.22857143 0.24285714 0.25714286 0.27142857 0.28571429 0.3 0.31428571 0.32857143 0.34285714 0.35714286 0.37142857 0.38571429 0.4 0.41428571 0.42857143 0.44285714 0.45714286 0.47142857 0.48571429 0.5 0.51428571 0.52857143 0.54285714 0.55714286 0.57142857 0.58571429 0.6 0.61428571 0.62857143 0.64285714 0.65714286 0.67142857 0.68571429 0.7 0.71428571 0.72857143 0.74285714 0.75714286 0.77142857 0.78571429 0.8 0.81428571 0.82857143 0.84285714 0.85714286 0.87142857 0.88571429 0.9 0.91428571 0.92857143 0.94285714 0.95714286 0.97142857 0.98571429 1 1 1 1 1 1
  arc A46 (13.5923, 28.4165) -> (11.7009, 29.2462) centre (0, 0) ccw
  spline S23 degree 5 poles (8.3174, 25.4569) (8.3217, 25.4702) (8.3307, 25.4965) (8.3453, 25.5357) (8.3667, 25.587) (8.3962, 25.6502) (8.4277, 25.7126) (8.4604, 25.7745) (8.4938, 25.8362) (8.5276, 25.8977) (8.5619, 25.959) (8.5968, 26.0201) (8.6325, 26.0808) (8.6691, 26.1411) (8.7067, 26.201) (8.7452, 26.2606) (8.7844, 26.3198) (8.8243, 26.3787) (8.8646, 26.4374) (8.9055, 26.4958) (8.9469, 26.554) (8.9889, 26.6119) (9.0314, 26.6696) (9.0745, 26.727) (9.1181, 26.7841) (9.1623, 26.841) (9.207, 26.8975) (9.2522, 26.9539) (9.2979, 27.01) (9.3441, 27.0658) (9.3907, 27.1214) (9.4377, 27.1768) (9.4853, 27.2319) (9.5332, 27.2868) (9.5816, 27.3415) (9.6305, 27.3959) (9.6798, 27.45) (9.7295, 27.5039) (9.7796, 27.5576) (9.8302, 27.6111) (9.8811, 27.6643) (9.9324, 27.7173) (9.9842, 27.77) (10.0363, 27.8226) (10.0888, 27.8749) (10.1417, 27.9269) (10.1949, 27.9788) (10.2486, 28.0303) (10.3026, 28.0817) (10.357, 28.1329) (10.4117, 28.1838) (10.4668, 28.2345) (10.5223, 28.2849) (10.5781, 28.3351) (10.6342, 28.3851) (10.6907, 28.4349) (10.7475, 28.4844) (10.8047, 28.5338) (10.8622, 28.5828) (10.92, 28.6317) (10.9782, 28.6803) (11.0367, 28.7287) (11.0955, 28.7769) (11.1546, 28.8249) (11.2141, 28.8726) (11.2739, 28.9201) (11.3339, 28.9674) (11.3943, 29.0144) (11.455, 29.0612) (11.516, 29.1078) (11.5773, 29.1542) (11.6266, 29.1911) (11.6637, 29.2187) (11.6885, 29.237) (11.7009, 29.2462) knots 0 0 0 0 0 0 0.01428571 0.02857143 0.04285714 0.05714286 0.07142857 0.08571429 0.1 0.11428571 0.12857143 0.14285714 0.15714286 0.17142857 0.18571429 0.2 0.21428571 0.22857143 0.24285714 0.25714286 0.27142857 0.28571429 0.3 0.31428571 0.32857143 0.34285714 0.35714286 0.37142857 0.38571429 0.4 0.41428571 0.42857143 0.44285714 0.45714286 0.47142857 0.48571429 0.5 0.51428571 0.52857143 0.54285714 0.55714286 0.57142857 0.58571429 0.6 0.61428571 0.62857143 0.64285714 0.65714286 0.67142857 0.68571429 0.7 0.71428571 0.72857143 0.74285714 0.75714286 0.77142857 0.78571429 0.8 0.81428571 0.82857143 0.84285714 0.85714286 0.87142857 0.88571429 0.9 0.91428571 0.92857143 0.94285714 0.95714286 0.97142857 0.98571429 1 1 1 1 1 1
  line L23 (8.3174, 25.4569) -> (8.0213, 24.5523)
  arc A47 (6.7973, 23.9014) -> (8.0213, 24.5523) centre (7.0709, 24.8633) ccw
  arc A48 (6.7973, 23.9014) -> (5.3977, 24.2559) centre (0, 0) ccw
  arc A49 (4.6311, 25.4108) -> (5.3977, 24.2559) centre (5.615, 25.232) ccw
  line L24 (4.6311, 25.4108) -> (4.8013, 26.3473)
  spline S24 degree 5 poles (4.8013, 26.3473) (4.8037, 26.3611) (4.8084, 26.3885) (4.8142, 26.4299) (4.8198, 26.4852) (4.8239, 26.5548) (4.8259, 26.6247) (4.8266, 26.6947) (4.8266, 26.7648) (4.8262, 26.835) (4.8252, 26.9052) (4.8236, 26.9756) (4.8211, 27.046) (4.8175, 27.1165) (4.813, 27.1871) (4.8075, 27.2577) (4.8012, 27.3285) (4.7942, 27.3992) (4.7866, 27.4701) (4.7784, 27.5409) (4.7697, 27.6118) (4.7604, 27.6827) (4.7505, 27.7537) (4.7399, 27.8247) (4.7287, 27.8957) (4.7169, 27.9667) (4.7045, 28.0377) (4.6915, 28.1088) (4.678, 28.1799) (4.664, 28.251) (4.6495, 28.3221) (4.6345, 28.3932) (4.6189, 28.4643) (4.6029, 28.5354) (4.5863, 28.6065) (4.5692, 28.6775) (4.5516, 28.7486) (4.5336, 28.8197) (4.5151, 28.8908) (4.4961, 28.9619) (4.4766, 29.0329) (4.4567, 29.1039) (4.4363, 29.175) (4.4154, 29.246) (4.3941, 29.3169) (4.3724, 29.3879) (4.3502, 29.4588) (4.3276, 29.5297) (4.3046, 29.6006) (4.2811, 29.6715) (4.2572, 29.7423) (4.2328, 29.8131) (4.2081, 29.8839) (4.1829, 29.9546) (4.1573, 30.0253) (4.1313, 30.096) (4.1049, 30.1666) (4.0781, 30.2372) (4.0509, 30.3077) (4.0233, 30.3782) (3.9953, 30.4487) (3.9669, 30.5191) (3.9381, 30.5894) (3.9089, 30.6597) (3.8793, 30.73) (3.8494, 30.8002) (3.819, 30.8704) (3.7883, 30.9405) (3.7572, 31.0106) (3.7258, 31.0806) (3.6939, 31.1505) (3.6681, 31.2065) (3.6486, 31.2484) (3.6355, 31.2763) (3.629, 31.2903) knots 0 0 0 0 0 0 0.01428571 0.02857143 0.04285714 0.05714286 0.07142857 0.08571429 0.1 0.11428571 0.12857143 0.14285714 0.15714286 0.17142857 0.18571429 0.2 0.21428571 0.22857143 0.24285714 0.25714286 0.27142857 0.28571429 0.3 0.31428571 0.32857143 0.34285714 0.35714286 0.37142857 0.38571429 0.4 0.41428571 0.42857143 0.44285714 0.45714286 0.47142857 0.48571429 0.5 0.51428571 0.52857143 0.54285714 0.55714286 0.57142857 0.58571429 0.6 0.61428571 0.62857143 0.64285714 0.65714286 0.67142857 0.68571429 0.7 0.71428571 0.72857143 0.74285714 0.75714286 0.77142857 0.78571429 0.8 0.81428571 0.82857143 0.84285714 0.85714286 0.87142857 0.88571429 0.9 0.91428571 0.92857143 0.94285714 0.95714286 0.97142857 0.98571429 1 1 1 1 1 1
  arc A50 (3.629, 31.2903) -> (1.5707, 31.4608) centre (0, 0) ccw
  spline S25 degree 5 poles (-0.3991, 26.7783) (-0.3993, 26.7922) (-0.3994, 26.8201) (-0.3983, 26.8618) (-0.3947, 26.9173) (-0.3873, 26.9866) (-0.3778, 27.0559) (-0.367, 27.125) (-0.3554, 27.1942) (-0.3434, 27.2634) (-0.3309, 27.3325) (-0.3177, 27.4016) (-0.3037, 27.4706) (-0.2886, 27.5396) (-0.2725, 27.6084) (-0.2554, 27.6772) (-0.2376, 27.746) (-0.219, 27.8146) (-0.1999, 27.8833) (-0.1802, 27.9518) (-0.1599, 28.0203) (-0.1391, 28.0887) (-0.1176, 28.1571) (-0.0955, 28.2253) (-0.0727, 28.2935) (-0.0494, 28.3616) (-0.0255, 28.4297) (-0.001, 28.4976) (0.024, 28.5655) (0.0495, 28.6333) (0.0755, 28.7011) (0.1021, 28.7687) (0.1291, 28.8363) (0.1567, 28.9038) (0.1847, 28.9712) (0.2133, 29.0385) (0.2423, 29.1057) (0.2718, 29.1729) (0.3018, 29.2399) (0.3322, 29.3069) (0.3631, 29.3738) (0.3945, 29.4405) (0.4263, 29.5072) (0.4585, 29.5738) (0.4912, 29.6403) (0.5243, 29.7068) (0.5579, 29.7731) (0.5919, 29.8393) (0.6263, 29.9054) (0.6611, 29.9714) (0.6963, 30.0374) (0.732, 30.1032) (0.768, 30.1689) (0.8045, 30.2345) (0.8414, 30.3001) (0.8786, 30.3655) (0.9163, 30.4308) (0.9544, 30.496) (0.9928, 30.5611) (1.0317, 30.6261) (1.0709, 30.691) (1.1105, 30.7558) (1.1505, 30.8204) (1.1908, 30.885) (1.2316, 30.9494) (1.2727, 31.0137) (1.3141, 31.078) (1.356, 31.1421) (1.3982, 31.2061) (1.4408, 31.2699) (1.4837, 31.3337) (1.5183, 31.3846) (1.5445, 31.4227) (1.5619, 31.4481) (1.5707, 31.4608) knots 0 0 0 0 0 0 0.01428571 0.02857143 0.04285714 0.05714286 0.07142857 0.08571429 0.1 0.11428571 0.12857143 0.14285714 0.15714286 0.17142857 0.18571429 0.2 0.21428571 0.22857143 0.24285714 0.25714286 0.27142857 0.28571429 0.3 0.31428571 0.32857143 0.34285714 0.35714286 0.37142857 0.38571429 0.4 0.41428571 0.42857143 0.44285714 0.45714286 0.47142857 0.48571429 0.5 0.51428571 0.52857143 0.54285714 0.55714286 0.57142857 0.58571429 0.6 0.61428571 0.62857143 0.64285714 0.65714286 0.67142857 0.68571429 0.7 0.71428571 0.72857143 0.74285714 0.75714286 0.77142857 0.78571429 0.8 0.81428571 0.82857143 0.84285714 0.85714286 0.87142857 0.88571429 0.9 0.91428571 0.92857143 0.94285714 0.95714286 0.97142857 0.98571429 1 1 1 1 1 1
  line L25 (-0.3991, 26.7783) -> (-0.3854, 25.8265)
  arc A51 (-1.3317, 24.8135) -> (-0.3854, 25.8265) centre (-1.3853, 25.8121) ccw
  arc A52 (-1.3317, 24.8135) -> (-2.7706, 24.6943) centre (0, 0) ccw
  arc A53 (-3.8707, 25.5377) -> (-2.7706, 24.6943) centre (-2.8821, 25.688) ccw
  line L26 (-3.8707, 25.5377) -> (-4.0139, 26.4787)
  spline S26 degree 5 poles (-4.0139, 26.4787) (-4.016, 26.4925) (-4.0205, 26.52) (-4.0285, 26.561) (-4.0411, 26.6152) (-4.0598, 26.6823) (-4.0806, 26.749) (-4.1027, 26.8155) (-4.1254, 26.8818) (-4.1486, 26.9481) (-4.1724, 27.0142) (-4.1967, 27.0802) (-4.222, 27.1459) (-4.2482, 27.2115) (-4.2754, 27.2767) (-4.3036, 27.3418) (-4.3325, 27.4067) (-4.3621, 27.4713) (-4.3923, 27.5359) (-4.423, 27.6002) (-4.4543, 27.6644) (-4.4861, 27.7285) (-4.5185, 27.7924) (-4.5516, 27.8561) (-4.5852, 27.9196) (-4.6195, 27.9829) (-4.6543, 28.0461) (-4.6896, 28.1091) (-4.7254, 28.172) (-4.7617, 28.2347) (-4.7986, 28.2972) (-4.8359, 28.3596) (-4.8737, 28.4217) (-4.9119, 28.4838) (-4.9507, 28.5456) (-4.9899, 28.6073) (-5.0297, 28.6689) (-5.0698, 28.7302) (-5.1104, 28.7915) (-5.1515, 28.8525) (-5.1929, 28.9134) (-5.2348, 28.9741) (-5.2772, 29.0346) (-5.32, 29.095) (-5.3631, 29.1552) (-5.4067, 29.2153) (-5.4508, 29.2752) (-5.4952, 29.3349) (-5.54, 29.3945) (-5.5852, 29.4539) (-5.6308, 29.5131) (-5.6768, 29.5722) (-5.7232, 29.631) (-5.77, 29.6898) (-5.8171, 29.7483) (-5.8647, 29.8067) (-5.9126, 29.8649) (-5.9608, 29.923) (-6.0095, 29.9809) (-6.0585, 30.0386) (-6.1078, 30.0961) (-6.1576, 30.1535) (-6.2077, 30.2107) (-6.2581, 30.2677) (-6.3089, 30.3246) (-6.36, 30.3813) (-6.4115, 30.4378) (-6.4633, 30.4941) (-6.5155, 30.5503) (-6.568, 30.6063) (-6.6208, 30.6621) (-6.6633, 30.7066) (-6.6954, 30.74) (-6.7168, 30.7621) (-6.7276, 30.7732) knots 0 0 0 0 0 0 0.01428571 0.02857143 0.04285714 0.05714286 0.07142857 0.08571429 0.1 0.11428571 0.12857143 0.14285714 0.15714286 0.17142857 0.18571429 0.2 0.21428571 0.22857143 0.24285714 0.25714286 0.27142857 0.28571429 0.3 0.31428571 0.32857143 0.34285714 0.35714286 0.37142857 0.38571429 0.4 0.41428571 0.42857143 0.44285714 0.45714286 0.47142857 0.48571429 0.5 0.51428571 0.52857143 0.54285714 0.55714286 0.57142857 0.58571429 0.6 0.61428571 0.62857143 0.64285714 0.65714286 0.67142857 0.68571429 0.7 0.71428571 0.72857143 0.74285714 0.75714286 0.77142857 0.78571429 0.8 0.81428571 0.82857143 0.84285714 0.85714286 0.87142857 0.88571429 0.9 0.91428571 0.92857143 0.94285714 0.95714286 0.97142857 0.98571429 1 1 1 1 1 1
  arc A54 (-6.7276, 30.7732) -> (-8.7297, 30.2662) centre (0, 0) ccw
  spline S27 degree 5 poles (-9.0724, 25.1977) (-9.0771, 25.2109) (-9.0862, 25.2372) (-9.0987, 25.277) (-9.1134, 25.3307) (-9.1289, 25.3987) (-9.1423, 25.4672) (-9.1546, 25.5362) (-9.1661, 25.6053) (-9.1772, 25.6746) (-9.1878, 25.7441) (-9.1978, 25.8137) (-9.2069, 25.8836) (-9.215, 25.9537) (-9.2222, 26.0241) (-9.2284, 26.0947) (-9.2338, 26.1655) (-9.2385, 26.2365) (-9.2427, 26.3076) (-9.2463, 26.3788) (-9.2494, 26.4502) (-9.2519, 26.5216) (-9.2538, 26.5932) (-9.255, 26.665) (-9.2557, 26.7369) (-9.2557, 26.8089) (-9.2552, 26.881) (-9.2541, 26.9532) (-9.2525, 27.0256) (-9.2504, 27.098) (-9.2478, 27.1705) (-9.2446, 27.2431) (-9.241, 27.3158) (-9.2369, 27.3886) (-9.2322, 27.4614) (-9.2271, 27.5344) (-9.2214, 27.6074) (-9.2153, 27.6805) (-9.2087, 27.7536) (-9.2017, 27.8268) (-9.1942, 27.9001) (-9.1862, 27.9735) (-9.1778, 28.0469) (-9.1689, 28.1203) (-9.1596, 28.1938) (-9.1499, 28.2674) (-9.1397, 28.341) (-9.129, 28.4147) (-9.1179, 28.4884) (-9.1064, 28.5622) (-9.0945, 28.636) (-9.0822, 28.7098) (-9.0694, 28.7837) (-9.0562, 28.8576) (-9.0426, 28.9315) (-9.0286, 29.0055) (-9.0142, 29.0795) (-8.9994, 29.1535) (-8.9841, 29.2276) (-8.9685, 29.3017) (-8.9525, 29.3758) (-8.9361, 29.4499) (-8.9192, 29.524) (-8.902, 29.5982) (-8.8844, 29.6724) (-8.8664, 29.7466) (-8.8481, 29.8208) (-8.8293, 29.895) (-8.8102, 29.9692) (-8.7906, 30.0434) (-8.7707, 30.1177) (-8.7545, 30.1771) (-8.7422, 30.2216) (-8.7339, 30.2513) (-8.7297, 30.2662) knots 0 0 0 0 0 0 0.01428571 0.02857143 0.04285714 0.05714286 0.07142857 0.08571429 0.1 0.11428571 0.12857143 0.14285714 0.15714286 0.17142857 0.18571429 0.2 0.21428571 0.22857143 0.24285714 0.25714286 0.27142857 0.28571429 0.3 0.31428571 0.32857143 0.34285714 0.35714286 0.37142857 0.38571429 0.4 0.41428571 0.42857143 0.44285714 0.45714286 0.47142857 0.48571429 0.5 0.51428571 0.52857143 0.54285714 0.55714286 0.57142857 0.58571429 0.6 0.61428571 0.62857143 0.64285714 0.65714286 0.67142857 0.68571429 0.7 0.71428571 0.72857143 0.74285714 0.75714286 0.77142857 0.78571429 0.8 0.81428571 0.82857143 0.84285714 0.85714286 0.87142857 0.88571429 0.9 0.91428571 0.92857143 0.94285714 0.95714286 0.97142857 0.98571429 1 1 1 1 1 1
  line L27 (-9.0724, 25.1977) -> (-8.7504, 24.302)
  arc A55 (-9.3165, 23.0366) -> (-8.7504, 24.302) centre (-9.6914, 23.9637) ccw
  arc A56 (-9.3165, 23.0366) -> (-10.6387, 22.4566) centre (0, 0) ccw
  arc A57 (-11.9531, 22.8971) -> (-10.6387, 22.4566) centre (-11.0668, 23.3604) ccw
  line L28 (-11.9531, 22.8971) -> (-12.394, 23.7408)
  spline S28 degree 5 poles (-12.394, 23.7408) (-12.4005, 23.7531) (-12.4137, 23.7776) (-12.4345, 23.8138) (-12.4641, 23.8609) (-12.5036, 23.9184) (-12.5449, 23.9747) (-12.5874, 24.0304) (-12.6304, 24.0858) (-12.6739, 24.1409) (-12.7178, 24.1957) (-12.7623, 24.2502) (-12.8075, 24.3042) (-12.8536, 24.3577) (-12.9005, 24.4106) (-12.9483, 24.463) (-12.9967, 24.5149) (-13.0457, 24.5665) (-13.0952, 24.6177) (-13.1451, 24.6686) (-13.1955, 24.7192) (-13.2465, 24.7695) (-13.2979, 24.8194) (-13.3498, 24.8689) (-13.4023, 24.918) (-13.4552, 24.9668) (-13.5086, 25.0153) (-13.5625, 25.0634) (-13.6168, 25.1112) (-13.6715, 25.1587) (-13.7266, 25.2059) (-13.7822, 25.2528) (-13.8381, 25.2993) (-13.8945, 25.3455) (-13.9512, 25.3915) (-14.0084, 25.4371) (-14.0659, 25.4824) (-14.1238, 25.5274) (-14.1821, 25.5721) (-14.2407, 25.6165) (-14.2997, 25.6606) (-14.3591, 25.7044) (-14.4188, 25.748) (-14.4788, 25.7912) (-14.5392, 25.8341) (-14.6, 25.8768) (-14.6611, 25.9191) (-14.7225, 25.9612) (-14.7842, 26.003) (-14.8462, 26.0445) (-14.9086, 26.0857) (-14.9713, 26.1266) (-15.0343, 26.1672) (-15.0976, 26.2076) (-15.1612, 26.2477) (-15.2251, 26.2875) (-15.2893, 26.327) (-15.3538, 26.3662) (-15.4186, 26.4052) (-15.4837, 26.4438) (-15.5491, 26.4822) (-15.6148, 26.5203) (-15.6807, 26.5582) (-15.7469, 26.5957) (-15.8134, 26.633) (-15.8802, 26.6701) (-15.9472, 26.7068) (-16.0145, 26.7433) (-16.0821, 26.7794) (-16.1499, 26.8154) (-16.218, 26.851) (-16.2727, 26.8793) (-16.3139, 26.9004) (-16.3413, 26.9144) (-16.3551, 26.9214) knots 0 0 0 0 0 0 0.01428571 0.02857143 0.04285714 0.05714286 0.07142857 0.08571429 0.1 0.11428571 0.12857143 0.14285714 0.15714286 0.17142857 0.18571429 0.2 0.21428571 0.22857143 0.24285714 0.25714286 0.27142857 0.28571429 0.3 0.31428571 0.32857143 0.34285714 0.35714286 0.37142857 0.38571429 0.4 0.41428571 0.42857143 0.44285714 0.45714286 0.47142857 0.48571429 0.5 0.51428571 0.52857143 0.54285714 0.55714286 0.57142857 0.58571429 0.6 0.61428571 0.62857143 0.64285714 0.65714286 0.67142857 0.68571429 0.7 0.71428571 0.72857143 0.74285714 0.75714286 0.77142857 0.78571429 0.8 0.81428571 0.82857143 0.84285714 0.85714286 0.87142857 0.88571429 0.9 0.91428571 0.92857143 0.94285714 0.95714286 0.97142857 0.98571429 1 1 1 1 1 1
  arc A58 (-16.3551, 26.9214) -> (-18.0841, 25.7918) centre (0, 0) ccw
  spline S29 degree 5 poles (-16.7625, 20.8867) (-16.7712, 20.8975) (-16.7884, 20.9195) (-16.8132, 20.9531) (-16.8444, 20.9991) (-16.8812, 21.0584) (-16.9162, 21.1188) (-16.9501, 21.1801) (-16.9835, 21.2417) (-17.0165, 21.3037) (-17.0491, 21.3659) (-17.0811, 21.4285) (-17.1124, 21.4916) (-17.1429, 21.5553) (-17.1725, 21.6196) (-17.2013, 21.6843) (-17.2294, 21.7496) (-17.2569, 21.8151) (-17.284, 21.881) (-17.3105, 21.9472) (-17.3366, 22.0137) (-17.3622, 22.0805) (-17.3872, 22.1476) (-17.4117, 22.2151) (-17.4356, 22.2829) (-17.459, 22.351) (-17.482, 22.4194) (-17.5044, 22.488) (-17.5264, 22.557) (-17.5479, 22.6261) (-17.5689, 22.6956) (-17.5896, 22.7653) (-17.6097, 22.8352) (-17.6294, 22.9054) (-17.6487, 22.9758) (-17.6675, 23.0464) (-17.6859, 23.1173) (-17.7038, 23.1884) (-17.7214, 23.2598) (-17.7385, 23.3313) (-17.7552, 23.4031) (-17.7715, 23.475) (-17.7873, 23.5472) (-17.8028, 23.6195) (-17.8179, 23.6921) (-17.8325, 23.7649) (-17.8468, 23.8378) (-17.8606, 23.9109) (-17.8741, 23.9842) (-17.8872, 24.0577) (-17.8998, 24.1314) (-17.9121, 24.2052) (-17.924, 24.2793) (-17.9356, 24.3534) (-17.9467, 24.4278) (-17.9575, 24.5023) (-17.9679, 24.577) (-17.9779, 24.6518) (-17.9875, 24.7268) (-17.9968, 24.8019) (-18.0057, 24.8772) (-18.0142, 24.9527) (-18.0224, 25.0283) (-18.0302, 25.104) (-18.0376, 25.1799) (-18.0447, 25.2559) (-18.0514, 25.332) (-18.0578, 25.4083) (-18.0638, 25.4847) (-18.0694, 25.5613) (-18.0747, 25.638) (-18.0786, 25.6994) (-18.0814, 25.7456) (-18.0832, 25.7764) (-18.0841, 25.7918) knots 0 0 0 0 0 0 0.01428571 0.02857143 0.04285714 0.05714286 0.07142857 0.08571429 0.1 0.11428571 0.12857143 0.14285714 0.15714286 0.17142857 0.18571429 0.2 0.21428571 0.22857143 0.24285714 0.25714286 0.27142857 0.28571429 0.3 0.31428571 0.32857143 0.34285714 0.35714286 0.37142857 0.38571429 0.4 0.41428571 0.42857143 0.44285714 0.45714286 0.47142857 0.48571429 0.5 0.51428571 0.52857143 0.54285714 0.55714286 0.57142857 0.58571429 0.6 0.61428571 0.62857143 0.64285714 0.65714286 0.67142857 0.68571429 0.7 0.71428571 0.72857143 0.74285714 0.75714286 0.77142857 0.78571429 0.8 0.81428571 0.82857143 0.84285714 0.85714286 0.87142857 0.88571429 0.9 0.91428571 0.92857143 0.94285714 0.95714286 0.97142857 0.98571429 1 1 1 1 1 1
  line L29 (-16.7625, 20.8867) -> (-16.1671, 20.144)
  arc A59 (-16.2917, 18.7634) -> (-16.1671, 20.144) centre (-16.9473, 19.5184) ccw
  arc A60 (-16.2917, 18.7634) -> (-17.3539, 17.7855) centre (0, 0) ccw